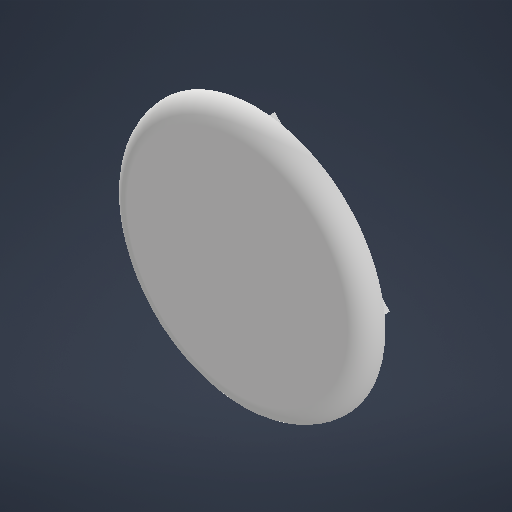
# Autodesk Inventor part: Part10
Saved by Autodesk Inventor 2026 (Build 300175000, 175)
## iProperties
Created: 2025-10-26
Part Number: Part10
Material: 一般
Document SubType Name: Modeling
Designer: masak
Density: 1 g/cm^3
Appearance: 既定
Author: masak
Autodesk Inventor part; units mm, degrees
ref_plane "YZ Plane" through (0, 0, 0) normal (1, 0, 0) x (0, 1, 0)
ref_plane "XZ Plane" through (0, 0, 0) normal (0, 1, 0) x (-1, 0, 0)
ref_plane "XY Plane" through (0, 0, 0) normal (0, 0, 1) x (1, 0, 0)
sketch "スケッチ1" plane through (0, 0, 0) normal (0, 0, 1) x (1, 0, 0)
  line L0 (23, 24.5) -> (3, 24.5) projected
  line L1 (23, 24.5) -> (3, 24.5) construction
  line L2 (23, 24.5) -> (3, 24.5)
  line L3 (23, 24.5) -> (3, 24.5)
  line L4 (23, 24.5) -> (3, 24.5)
  line L5 (23, 24.5) -> (3, 24.5) construction
  line L6 (13, 14.5) -> (3, 24.5) projected
  line L7 (3, 1.5) -> (13, 11.5) projected
  line L8 (11.5, 13) -> (1.5, 3) projected
  line L9 (1.5, 23) -> (11.5, 13) projected
  line L10 (1.5, 3) -> (1.5, 23) projected
  line L11 (0, 0) -> (0, 26) projected
  line L12 (0, 26) -> (50.5, 26) projected
  line L13 (50.5, 0) -> (0, 0) projected
  line L14 (0, 0) -> (-26, 0)
  line L15 (-26, 0) -> (-26, 26)
  line L16 (-26, 26) -> (0, 26)
  line L17 (0, 26) -> (0, 0)
  line L18 (-26, 0) -> (0, 26)
  line L19 (0, 0) -> (-26, 26)
  circle A0 centre (-13, 13) radius 27.5
  dimension "d0" = 26
  constraints: 18 end point, 2 parallel, 2 perpendicular, 1 centre point, 1 coincident, 1 horizontal, 1 midpoint
  measures "d0" distance of L15.end L16.end
extrude "押し出し1" add sketch "スケッチ1" along normal blind 4 contours L8 L10 L9 | L19 L18 L11 | L11 L12 A0 L13 | L13 A0 L12 L16 L15 L14 | L14 L18 L19 | L18 L19 L16 | L15 L19 L18
sketch "スケッチ2" plane through (-13, 13, 0) normal (0, 0, -1) x (-1, 0, 0)
  line L0 (-24.5, 0) -> (-14.5, 10) projected
  line L1 (-14.5, 10) -> (-14.5, -10) projected
  line L2 (-14.5, -10) -> (-24.5, 0) projected
  line L3 (-14.5, 10) -> (-14.5, -10)
  line L4 (-24.5, 0) -> (-14.5, 10)
  line L5 (-24.5, 0) -> (-14.5, -10)
  line L6 (-10, -14.5) -> (10, -14.5)
  line L7 (0, -24.5) -> (-10, -14.5)
  line L8 (0, -24.5) -> (10, -14.5)
  line L9 (14.5, -10) -> (14.5, 10)
  line L10 (24.5, 0) -> (14.5, -10)
  line L11 (24.5, 0) -> (14.5, 10)
  line L12 (10, 14.5) -> (-10, 14.5)
  line L13 (0, 24.5) -> (10, 14.5)
  line L14 (0, 24.5) -> (-10, 14.5)
  point P0 (-13, -13)
  point P1 (0, 0)
  dimension "d5" = 360
  constraints: 24 end point, 1 perpendicular, 1 vertical, 25 other
fillet "フィレット1" radius 4 1 edges at (-40.5, 13, 4)
extrude "押し出し2" add sketch "スケッチ2" along normal blind 4
